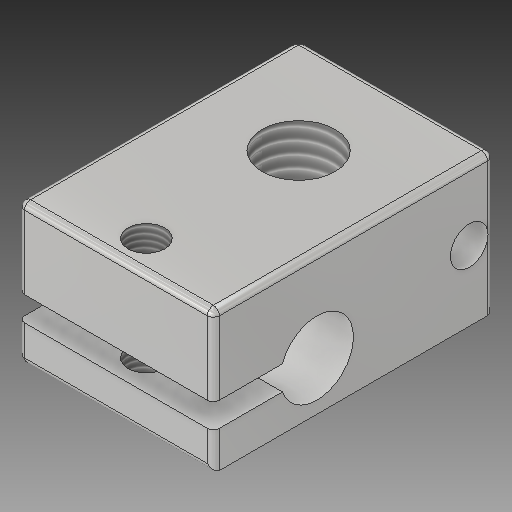
# Autodesk Inventor part: E3Dv6_Heater_Block
Saved by Autodesk Inventor 2019 (Build 230136000, 136)
## iProperties
Created: 2018-10-04
Part Number: E3Dv6_Heater_Block
Material: Generic
Document SubType Name: Modeling
Designer: Ax
Density: 1 g/cm^3
Appearance: Default
Author: Ax
Autodesk Inventor part; units mm, degrees
ref_plane "YZ Plane" through (0, 0, 0) normal (1, 0, 0) x (0, 1, 0)
ref_plane "XZ Plane" through (0, 0, 0) normal (0, 1, 0) x (-1, 0, 0)
ref_plane "XY Plane" through (0, 0, 0) normal (0, 0, 1) x (1, 0, 0)
sketch "Sketch1" plane through (0, 0, 0) normal (0, 1, 0) x (-1, 0, 0)
  line L0 (-8, 11.5) -> (8, 11.5)
  line L1 (8, 11.5) -> (8, -11.5)
  line L2 (8, -11.5) -> (-8, -11.5)
  line L3 (-8, -11.5) -> (-8, 11.5)
  line L4 (-8, 11.5) -> (8, -11.5) construction
  line L5 (8, 11.5) -> (-8, -11.5) construction
  point P0 (0, 0)
  dimension "d0" = 16
  dimension "d1" = 23
  constraints: 12 end point, 2 midpoint, 2 parallel, 1 horizontal, 1 perpendicular
  measures "d0" distance of L1.end L2.end
  measures "d1" distance of L0.end L1.end
extrude "Extrusion1" add sketch "Sketch1" along normal blind 11.5
sketch "Sketch2" plane through (8, 0, 11.5) normal (1, 0, 0) x (0, 0, -1)
  arc A0 (5.6716, 3) -> (5.6716, 5) centre (8.5, 4) ccw
  line L0 (23, 0) -> (23, 11.5) projected
  line L1 (23, 0) -> (0, 0) projected
  line L2 (0, 5) -> (5.6716, 5)
  line L3 (0, 5) -> (0, 3)
  line L4 (0, 0) -> (0, 11.5) projected
  line L5 (0, 3) -> (5.6716, 3)
  line L6 (8.5, 4) -> (0, 4) construction
  circle A1 centre (21, 5.74) radius 1.55
  point P0 (11.5, 0)
  dimension "d4" = 14.5
  dimension "d5" = 6
  dimension "d6" = 4
  dimension "d7" = 8.5
  dimension "d8" = 2
  dimension "d9" = 3.1
  dimension "d10" = 2
  dimension "d11" = 5.74
  constraints: 8 end point, 2 centre point, 2 horizontal, 2 point on circle, 2 point on line, 1 perpendicular, 1 symmetric about line
  measures "d4" distance from line of L0 L6.start
  measures "d5" diameter of A0
  measures "d6" distance from line of L1 L6.start
  measures "d7" distance of L6.start L6.end
  measures "d8" distance of L2.start L3.end
  measures "d9" diameter of A1
  measures "d10" distance from line of L0 A1.centre
  measures "d11" distance from line of A1.centre L1
extrude "Extrusion2" cut sketch "Sketch2" against normal through all
sketch "Sketch3" plane through (0, 11.5, 0) normal (0, 1, 0) x (1, 0, 0)
  line L0 (8, -11.5) -> (-8, -11.5) construction
  line L1 (0, -11.5) -> (0, 11.545) construction
  circle A0 centre (0, 3.5) radius 3
  circle A1 centre (0, -9) radius 1.5
  line L2 (8, 11.5) -> (-8, 11.5) projected
  point P0 (0, 0)
  dimension "d14" = 8
  dimension "d15" = 6
  dimension "d17" = 20.5
  dimension "d18" = 3
  constraints: 2 centre point, 2 end point, 2 point on line, 1 midpoint, 1 vertical
  measures "d14" distance from line of L2 A0.centre
  measures "d15" diameter of A0
  measures "d17" distance from line of L2 A1.centre
  measures "d18" diameter of A1
extrude "Extrusion3" cut sketch "Sketch3" against normal through all
sketch "Sketch4" plane through (0, 0, 0) normal (0, -1, 0) x (1, 0, 0)
  line L0 (0, 0) -> (0, -11.4648) construction
  circle A0 centre (0, -9.5) radius 1.5
  line L1 (-8, -11.5) -> (8, -11.5) projected
  dimension "d21" = 3
  dimension "d22" = 2
  constraints: 2 end point, 1 centre point, 1 point on line, 1 vertical
  measures "d21" diameter of A0
  measures "d22" distance from line of L1 A0.centre
extrude "Extrusion4" cut sketch "Sketch4" against normal up to surface round surface about axis through (8, 5.74, -9.5) along (-1, 0, 0) radius 1.55 far side no
fillet "Fillet1" radius 0.5 13 edges at (8, 11.5, 0) (8, 5.75, -11.5) (-8, 5.75, -11.5) (0, 11.5, -11.5) (0, 0, -11.5) (-8, 0, 0) (-8, 11.5, 0) (8, 8.25, 11.5) (8, 1.5, 11.5) (-8, 1.5, 11.5) (-8, 8.25, 11.5) (0, 11.5, 11.5) (0, 0, 11.5)
thread "Thread1" size "M6x1" class "6H" standard "ISO Metric profile" full length
thread "Thread2" size "M3x0.5" class "6H" standard "ISO Metric profile" full length
thread "Thread3" size "M3x0.5" class "6H" standard "ANSI Metric M Profile" full length
thread "Thread4" size "M3x0.5" class "6H" standard "ANSI Metric M Profile" full length
body "Solid1"
